ROT_ENCODER (Autodesk Fusion 360 design; units mm, degrees)
Autodesk Fusion 360 part; units mm, degrees
sketch "Esquisse1" plane through (0, 0, 0) normal (0, 0, 1) x (1, 0, 0)
  line L0 (8, -16) -> (-8, -16)
  line L1 (-12, -12) -> (-12, 12)
  line L2 (-8, 16) -> (8, 16)
  line L3 (12, 12) -> (12, -12)
  line L4 (12, -16) -> (-12, 16) construction
  line L5 (-12, -16) -> (12, 16) construction
  circle A0 centre (-8, -4) radius 2.425
  circle A1 centre (8, -4) radius 2.425
  circle A2 centre (0, 8) radius 5
  arc A3 (-12, -12) -> (-8, -16) centre (-8, -12) ccw
  arc A4 (8, -16) -> (12, -12) centre (8, -12) ccw
  arc A5 (12, 12) -> (8, 16) centre (8, 12) ccw
  arc A6 (-8, 16) -> (-12, 12) centre (-8, 12) ccw
  dimension "d1" = 24
  dimension "d2" = 32
  dimension "d3" = 4.85
  dimension "d4" = 4.85
  dimension "d5" = 12
  dimension "d6" = 12
  dimension "d7" = 16
  dimension "d8" = 10
  dimension "d9" = 8
  dimension "d10" = 4
  constraint horizontal L0
  constraint perpendicular L0 L1
  constraint parallel L0 L2
  constraint parallel L1 L3
  constraint coincident L4 origin
  constraint coincident L5 origin
  constraint coincident L5.start L1
  constraint coincident L5.start L0
  constraint tangent L1 A3
  constraint tangent L0 A3
  constraint coincident L4.start L3
  constraint coincident L4.start L0
  constraint tangent L3 A4
  constraint tangent L0 A4
  constraint equal A3 A4
  constraint coincident L5.end L3
  constraint coincident L5.end L2
  constraint tangent L3 A5
  constraint tangent L2 A5
  constraint equal A3 A5
  constraint coincident L4.end L2
  constraint coincident L4.end L1
  constraint tangent L2 A6
  constraint tangent L1 A6
  constraint equal A3 A6
  measures "d1" distance of L4.end L5.end
  measures "d2" distance of L5.start L4.end
  measures "d3" diameter of A0
  measures "d4" diameter of A1
  measures "d5" distance of L0 A0.centre
  measures "d6" distance of L0 A1.centre
  measures "d7" distance of A0.centre A1.centre
  measures "d8" diameter of A2
  measures "d9" distance of L2 A2.centre
  measures "d10" radius of A3
extrude "Extrusion1" add sketch "Esquisse1" against normal blind 8 contours L0 L1 L2 L3 A3 A4 A5 A6 | A2
extrude "Extrusion2" add sketch "Esquisse1" along normal blind 25.4 contours A2
fillet "Congé1" radius 0.5 16 edges at (0, -16, -8) (-10.8284, -14.8284, -8) (-12, 0, -8) (-10.8284, 14.8284, -8) (0, 16, -8) (10.8284, 14.8284, -8) (12, 0, -8) (10.8284, -14.8284, -8) (10.8284, -14.8284, 0) (0, -16, 0) (-10.8284, -14.8284, 0) (-12, 0, 0) (-10.8284, 14.8284, 0) (0, 16, 0) (10.8284, 14.8284, 0) (12, 0, 0)
fillet "Congé2" radius 1.5 1 edges at (-4.6616, 6.1919, 25.4)
equation "d6 = d5"
